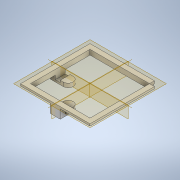
# Autodesk Inventor part: Marker_Edge
Saved by Autodesk Inventor 2022.4 (Build 264492010, 492A)
## iProperties
Created: 2025-03-21
Part Number: Marker_Edge
Material: Generic
Document SubType Name: Modeling
Designer: jan-m
Density: 1 g/cm^3
Appearance: Default
Author: jan-m
Autodesk Inventor part; units mm, degrees
sketch "Sketch1" plane through (0, 0, 0) normal (0, 1, 0) x (-1, 0, 0)
  line L0 (30, -30) -> (-30, -30)
  line L1 (-30, -30) -> (-30, 30)
  line L2 (-30, 30) -> (30, 30)
  line L3 (30, 30) -> (30, -30)
  line L4 (0, -49) -> (0, 49) projected
  line L5 (-49, 0) -> (49, 0) projected
  line L6 (-35, -35) -> (35, -35)
  line L7 (35, -35) -> (35, 35)
  line L8 (35, 35) -> (-35, 35)
  line L9 (-35, 35) -> (-35, -35)
  line L10 (-30, -30) -> (-30, -35)
  line L11 (-30, -30) -> (-35, -30)
  line L12 (-32, -32) -> (32, -32)
  line L13 (32, -32) -> (32, 32)
  line L14 (32, 32) -> (-32, 32)
  line L15 (-32, 32) -> (-32, -32)
  point P0 (0, 0)
  point P1 (0, -30)
  point P2 (30, 0)
  point P3 (-30, -32)
  point P4 (-32, -30)
  dimension "d0" = 60
  dimension "d1" = 60
  dimension "d2" = 5
  dimension "d3" = 2
  constraints: 28 end point, 6 parallel, 5 perpendicular, 4 point on line, 2 midpoint, 1 horizontal, 6 other
  measures "d0" distance of L0.start L0.end
  measures "d1" distance of L2.end L0.start
  measures "d2" distance between parallel lines of L0 L6
  measures "d3" distance between parallel lines of L0 L12
extrude "Extrusion1" add sketch "Sketch1" against normal blind 2 contours L12 L13 L5 L7 L6 L4 | L4 L6 L10 L12 | L13 L14 L4 L8 L7 L5 | L11 L9 L5 L15 | L5 L9 L8 L4 L14 L15
extrude "Extrusion2" add sketch "Sketch1" against normal blind 5 contours L3 L5 L13 L12 L4 L0 | L4 L12 L10 L0 | L3 L2 L4 L14 L13 L5 | L11 L15 L5 L1 | L5 L15 L14 L4 L2 L1
chamfer "Chamfer1" distance 3 angle 45 4 edges at (0, -2, 32) (32, -2, 1) (-1, -2, -32) (-32, -2, 0)
sketch "Sketch2" plane through (0, 0, 0) normal (0, 1, 0) x (1, 0, 0)
  line L0 (-30, -30) -> (30, -30) projected
  line L1 (-35, -35) -> (35, -35) projected
  line L2 (-5, -30) -> (5, -30)
  line L3 (5, -30) -> (5, -35)
  line L4 (5, -35) -> (-5, -35)
  line L5 (-5, -35) -> (-5, -30)
  line L6 (0, 49) -> (0, -49) projected
  point P0 (0, 0)
  point P1 (0, -35)
  dimension "d11" = 10
  constraints: 8 end point, 3 point on line, 2 parallel, 1 horizontal, 1 midpoint, 1 perpendicular
  measures "d11" distance between parallel lines of L3 L5
extrude "Extrusion3" add sketch "Sketch2" against normal blind 11
sketch "Sketch3" plane through (0, -11, 0) normal (0, -1, 0) x (1, 0, 0)
  line L0 (5, 30) -> (30, 30) projected
  line L1 (5, 30) -> (-5, 30)
  line L2 (-5, 30) -> (-5, 25)
  line L3 (-5, 25) -> (5, 25)
  line L4 (5, 25) -> (5, 30)
  line L5 (-5, 25) -> (5, 25)
  line L6 (5, 25) -> (5, 22)
  line L7 (5, 22) -> (-5, 22)
  line L8 (-5, 22) -> (-5, 25)
  arc A0 (-5, 22) -> (5, 22) centre (0, 22) ccw
  point P0 (0, 0)
  dimension "d14" = 10
  dimension "d15" = 5
  dimension "d16" = 10
  dimension "d17" = 3
  dimension "d18" = 5
  constraints: 16 end point, 4 parallel, 2 horizontal, 2 perpendicular, 2 point on circle, 1 centre point
  measures "d14" distance of L3.end L2.end
  measures "d15" distance of L2.end L1.end
  measures "d16" distance of L6.end L7.end
  measures "d17" distance of L5.end L6.end
  measures "d18" radius of A0
extrude "Extrusion4" add sketch "Sketch3" against normal blind 2 contours L4 L3 L2 L1
extrude "Extrusion5" add sketch "Sketch3" against normal blind 4 contours L6 L7 L8 L3 | A0 L7
pattern_circular "Circular Pattern1" count 2 over 90 about axis through (0, -10, 0) along (0, -1, 0) of "Extrusion3", "Extrusion4", "Extrusion5"
body "Solid1"
